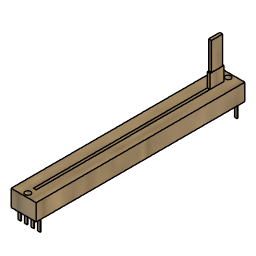
Pot-Slider-Final (Autodesk Fusion 360 design; units mm, degrees)
Autodesk Fusion 360 part; units mm, degrees
sketch "Skizze1" plane through (0, 0, 0) normal (0, 0, 1) x (1, 0, 0)
  line L0 (-4, 35) -> (5, 35)
  line L1 (5, 35) -> (5, -40)
  line L2 (5, -40) -> (-4, -40)
  line L3 (-4, -40) -> (-4, 35)
  line L4 (0, 31) -> (1, 31)
  line L5 (1, 31) -> (1, -36)
  line L6 (1, -36) -> (0, -36)
  line L7 (0, -36) -> (0, 31)
  line L8 (1, 27.3633) -> (0, 27.3633)
  line L9 (0, 27.3633) -> (0, 23.3633)
  line L10 (0, 23.3633) -> (1, 23.3633)
  line L11 (1, 23.3633) -> (1, 27.3633)
  circle A0 centre (0.5, -38.5) radius 1
  circle A1 centre (0.5, 33.5) radius 1
  dimension "d1" = 75
  dimension "d2" = 9
  dimension "d8" = 1
  dimension "d9" = 4
  dimension "d10" = 4
  dimension "d11" = 4
  dimension "d20" = 4
  dimension "d25" = 2
  dimension "d26" = 2.5
  dimension "d27" = 2
  dimension "d28" = 2.5
  constraint horizontal L0
  constraint vertical L1
  constraint horizontal L2
  constraint vertical L3
  constraint horizontal L4
  constraint vertical L5
  constraint horizontal L6
  constraint vertical L7
  constraint horizontal L8
  constraint vertical L9
  constraint horizontal L10
  constraint vertical L11
  constraint coincident L7 L9.end
  constraint coincident L5 L8.start
  measures "d1" distance of L0.end L1.end
  measures "d2" distance of L0.start L0.end
  measures "d8" distance of L5 L7
  measures "d9" distance of L1 L5
  measures "d10" distance of L2 L6
  measures "d11" distance of L0 L4
  measures "d20" distance of L8.start L10.end
  measures "d25" diameter of A0
  measures "d26" distance of L6 A0.centre
  measures "d27" diameter of A1
  measures "d28" distance of L4 A1.centre
extrude "Extrusion2" add sketch "Skizze1" along normal blind 6 contours L0 L1 L2 L3 | L4 L5 L7 L8 | L5 L7 L8 L9 L10 L11 | L5 L6 L7 L10 | A0 | A1 makes body 1
extrude "Extrusion3" cut sketch "Skizze1" along normal blind 5 contours L4 L5 L7 L8 | L5 L7 L8 L9 L10 L11 | L5 L6 L7 L10 bodies 1
extrude "Extrusion4" add sketch "Skizze1" along normal blind 6 separate body contours L4 L5 L7 L8 | L5 L7 L8 L9 L10 L11 | L5 L6 L7 L10 makes body 2
extrude "Extrusion5" cut 1 faces at (0.3333, -16.2122, 6) along direction (0, 0, -1) blind 1 on bodies 2 bodies 1 2
extrude "Extrusion7" add sketch "Skizze1" along normal blind 21 separate body contours L5 L7 L8 L9 L10 L11 makes body 3
extrude "Extrusion6" add sketch "Skizze1" along normal blind 22 contours L5 L7 L8 L9 L10 L11 bodies 1
delete_face "Fläche löschen1" 1 faces at (0.3333, 23.3633, 11.3333) on bodies 1
copy_body "Körper->Berechn1" bodies 3 removing the originals makes body 4 in component "slider"
move_body "Verschieben1" bodies 4 to x (1, 0, 0) y (0, 1, 0) z (0, 0, 1) at (0, 3.61, 0) in component "slider"
move_body "Verschieben2" bodies 4 to x (1, 0, 0) y (0, 1, 0) z (0, 0, 1) at (0, 0.02, 0) in component "slider"
extrude "Extrusion9" cut sketch "Skizze1" along normal blind 6 contours A1 bodies 1
extrude "Extrusion10" add sketch "Skizze1" along normal blind 1 contours A1 bodies 1
extrude "Extrusion11" cut sketch "Skizze1" along normal blind 2 contours A1 bodies 1
extrude "Extrusion12" add sketch "Skizze1" along normal blind 2 contours A1 bodies 1
extrude "Extrusion13" cut sketch "Skizze1" along normal blind 6 contours A0 bodies 1
extrude "Extrusion14" add sketch "Skizze1" along normal blind 2 contours A0 bodies 1
ref_plane "Arbeitsebene2" through (0.5, 28.9933, 11) normal (0, 0, 1) x (1, 0, 0)
sketch "Skizze5" plane through (0, 0, 11) normal (0, 0, 1) x (1, 0, 0)
  line L0 (0, 31.4933) -> (1.0088, 31.4933)
  line L1 (1.0088, 31.4933) -> (1.0088, 26.4933)
  line L2 (1.0088, 26.4933) -> (0, 26.4933)
  line L3 (0, 26.4933) -> (0, 31.4933)
  line L4 (1, 30.9933) -> (0, 30.9933)
  line L5 (0, 26.9933) -> (1, 26.9933)
  constraint horizontal L0
  constraint vertical L1
  constraint horizontal L2
  constraint vertical L3
extrude "Extrusion1" add sketch "Skizze5" against normal blind 5 bodies 4 in component "slider"
sketch "Skizze6" plane through (0, 0, 0) normal (0, 0, -1) x (1, 0, 0)
  line L0 (5, 40) -> (-4, 40)
  line L1 (-4, 40) -> (-4, -35)
  line L2 (-4, -35) -> (5, -35)
  line L3 (5, -35) -> (5, 40)
  line L4 (1, 36) -> (1, -31)
  line L5 (1, -31) -> (0, -31)
  line L6 (0, -31) -> (0, 36)
  line L7 (0, 36) -> (1, 36)
  line L8 (5, -33) -> (-4, -33)
  line L9 (-1, -33) -> (0, -33)
  line L10 (3.5, -33) -> (4.5, -33)
  line L11 (5, 38) -> (-4, 38)
  line L12 (4.5, 38) -> (3.5, 38)
  line L13 (3.5, 38) -> (3.5, 37.8)
  line L14 (3.5, 37.8) -> (4.5, 37.8)
  line L15 (4.5, 37.8) -> (4.5, 38)
  line L16 (-1, -33) -> (-1, -32.8)
  line L17 (-1, -32.8) -> (0, -32.8)
  line L18 (0, -32.8) -> (0, -33)
  line L19 (4.5, -33) -> (3.5, -33)
  line L20 (3.5, -33) -> (3.5, -32.8)
  line L21 (3.5, -32.8) -> (4.5, -32.8)
  line L22 (4.5, -32.8) -> (4.5, -33)
  line L23 (-3.5, 38) -> (-2.5, 38)
  line L24 (-2.5, 38) -> (-2.5, 37.8)
  line L25 (-2.5, 37.8) -> (-3.5, 37.8)
  line L26 (-3.5, 37.8) -> (-3.5, 38)
  line L27 (2.17, 38) -> (1.17, 38)
  line L28 (1.17, 38) -> (1.17, 37.8)
  line L29 (1.17, 37.8) -> (2.17, 37.8)
  line L30 (2.17, 37.8) -> (2.17, 38)
  line L31 (-0.16, 38) -> (-1.16, 38)
  line L32 (-1.16, 38) -> (-1.16, 37.8)
  line L33 (-1.16, 37.8) -> (-0.16, 37.8)
  line L34 (-0.16, 37.8) -> (-0.16, 38)
  dimension "d54" = 2
  dimension "d55" = 3
  dimension "d66" = 2
  dimension "d67" = 1
  dimension "d68" = 0.2
  dimension "d69" = 1
  dimension "d70" = 0.2
  dimension "d71" = 1
  dimension "d72" = 0.5
  dimension "d73" = 0.5
  dimension "d74" = 0.2
  dimension "d75" = 1
  dimension "d76" = 0.5
  dimension "d77" = 0.2
  dimension "d78" = 0.2
  dimension "d79" = 1
  dimension "d80" = 0.2
  dimension "d81" = 1
  dimension "d82" = 1.33
  dimension "d83" = 1.33
  dimension "d85" = 1.34
  constraint coincident L3 L8.start
  constraint coincident L1 L8.end
  constraint perpendicular L1 L8
  constraint horizontal L9
  constraint horizontal L10
  constraint coincident L8 L10.start
  constraint coincident L3 L11.start
  constraint coincident L1 L11.end
  constraint perpendicular L1 L11
  constraint horizontal L12
  constraint vertical L13
  constraint horizontal L14
  constraint vertical L15
  constraint coincident L11 L12.start
  constraint vertical L16
  constraint horizontal L17
  constraint vertical L18
  constraint horizontal L19
  constraint vertical L20
  constraint horizontal L21
  constraint vertical L22
  constraint horizontal L23
  constraint vertical L24
  constraint horizontal L25
  constraint vertical L26
  constraint coincident L11 L23.start
  constraint horizontal L27
  constraint vertical L28
  constraint horizontal L29
  constraint vertical L30
  constraint coincident L11 L27.start
  constraint horizontal L31
  constraint vertical L32
  constraint horizontal L33
  constraint vertical L34
  constraint coincident L11 L31.start
  measures "d54" distance of L2 L8
  measures "d55" distance of L8.end L9.start
  measures "d66" distance of L0 L11
  measures "d67" distance of L13.end L14.end
  measures "d68" distance of L9.end L17.end
  measures "d69" distance of L16.end L17.end
  measures "d70" distance of L10.start L20.end
  measures "d71" distance of L20.end L21.end
  measures "d72" distance of L3 L22
  measures "d73" distance of L3 L15
  measures "d74" distance of L23.start L25.end
  measures "d75" distance of L24.end L25.end
  measures "d76" distance of L1 L26
  measures "d77" distance of L12.end L13.end
  measures "d78" distance of L27.start L29.end
  measures "d79" distance of L28.end L29.end
  measures "d80" distance of L31.start L33.end
  measures "d81" distance of L32.end L33.end
  measures "d82" distance of L13 L30
  measures "d83" distance of L28 L34
  measures "d85" distance of L24 L32
extrude "Extrusion15" add sketch "Skizze6" along normal blind 4.5 contours L8 L9 L16 L17 L18 bodies 1
extrude "Extrusion16" add sketch "Skizze6" along normal blind 4.5 contours L8 L10 L19 L20 L21 L22 bodies 1
extrude "Extrusion17" add sketch "Skizze6" along normal blind 4.5 contours L11 L12 L13 L14 L15 | L11 L23 L24 L25 L26 | L11 L27 L28 L29 L30 | L11 L31 L32 L33 L34 bodies 1
sketch "Skizze7" plane through (0, 35, 0) normal (0, 1, 0) x (-1, 0, 0)
  line L0 (4, 6) -> (-5, 6)
  line L1 (-5, 6) -> (-5, 0)
  line L2 (-5, 0) -> (4, 0)
  line L3 (4, 0) -> (4, 6)
  line L4 (-4.9799, -0.0299) -> (4, 0) construction
  line L5 (4, 0) -> (3.9799, 6.0299) construction
  line L6 (3.9799, 6.0299) -> (-5, 6) construction
  line L7 (-5, 6) -> (-4.9799, -0.0299) construction
  dimension "d92" = 0.5
  text T0 "TOP" font "Arial" height 0.5 align centre middle in box 8.9799 x 6.03 at (-4.9799, -0.0299) x (0.999994, 0.003335) y (-0.003335, 0.999994) spacing 1 kerned
  constraint coincident L2.end
  constraint coincident L0.end
extrude "Extrusion18" cut sketch "Skizze7" against normal blind 0.1 text T0 bodies 1
extrude "Extrusion8" [suppressed]
component "slider" placed x (1, 0, 0) y (0, 1, 0) z (0, 0, 1) at (0, 0, 0)
equation "d21 = 6 mm + 16 mm"
named bodies: "Korpus", "MItte", "Silder"
